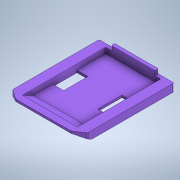
# Autodesk Inventor part: HullTop
Saved by Autodesk Inventor 2021 (Build 250183000, 183)
## iProperties
Created: 2021-05-14
Part Number: HullTop
Material: Generic
Document SubType Name: Modeling
Designer: ermoz
Density: 1 g/cm^3
Appearance: Default
Author: ermoz
Autodesk Inventor part; units mm, degrees
ref_plane "YZ Plane" through (0, 0, 0) normal (1, 0, 0) x (0, 1, 0)
ref_plane "XZ Plane" through (0, 0, 0) normal (0, 1, 0) x (-1, 0, 0)
ref_plane "XY Plane" through (0, 0, 0) normal (0, 0, 1) x (1, 0, 0)
sketch "Sketch1" plane through (0, 0, 0) normal (0, 1, 0) x (-1, 0, 0)
  line L0 (-34, 39.25) -> (34, 39.25)
  line L1 (34, 39.25) -> (34, -39.25)
  line L2 (34, -39.25) -> (-34, -39.25)
  line L3 (-34, -39.25) -> (-34, 39.25)
  line L4 (-34, 39.25) -> (34, -39.25) construction
  line L5 (34, 39.25) -> (-34, -39.25) construction
  line L6 (34, -39.25) -> (25, -39.25)
  line L7 (25, -39.25) -> (25, 39.25)
  line L8 (25, 39.25) -> (34, 39.25)
  line L9 (34, 39.25) -> (34, -39.25)
  line L10 (-34, -39.25) -> (-25, -39.25)
  line L11 (-25, -39.25) -> (-25, 39.25)
  line L12 (-25, 39.25) -> (-34, 39.25)
  line L13 (-34, 39.25) -> (-34, -39.25)
  circle A0 centre (29.5, 34.75) radius 1.5
  circle A1 centre (-29.5, 34.75) radius 1.5
  point P0 (0, 0)
  dimension "d0" = 78.5
  dimension "d1" = 68
  dimension "d2" = 9
  dimension "d3" = 9
  dimension "d4" = 3
  dimension "d5" = 4.5
  dimension "d6" = 3
  constraints: 28 end point, 6 parallel, 3 horizontal, 3 perpendicular, 2 centre point, 2 midpoint, 2 point on line
  measures "d0" distance of L0.end L1.end
  measures "d1" distance of L1.end L2.end
  measures "d2" distance of L7.end L8.end
  measures "d3" distance of L12.end L11.end
  measures "d4" diameter of A0
  measures "d5" distance from line of L0 A0.centre
  measures "d6" diameter of A1
extrude "Extrusion1" add sketch "Sketch1" along normal blind 2 contours L0 L7 L2 L11
extrude "Extrusion2" add sketch "Sketch1" along normal blind 7 contours L0 L11 L2 L3 | L0 L1 L2 L7 | A0 | A1
sketch "Sketch2" plane through (0, 2, 0) normal (0, 1, 0) x (1, 0, 0)
  line L0 (25, 39.25) -> (-25, 39.25) projected
  line L1 (-20, 39.25) -> (20, 39.25)
  line L2 (20, 39.25) -> (20, 36.25)
  line L3 (20, 36.25) -> (-20, 36.25)
  line L4 (-20, 36.25) -> (-20, 39.25)
  line L5 (25, 39.25) -> (25, -39.25) projected
  line L6 (-25, -39.25) -> (-25, 39.25) projected
  line L7 (-25, 39.25) -> (-20, 39.25)
  line L8 (-20, 39.25) -> (-20, 36.25)
  line L9 (-20, 36.25) -> (-25, 36.25)
  line L10 (-25, 36.25) -> (-25, 39.25)
  line L11 (20, 39.25) -> (25, 39.25)
  line L12 (25, 39.25) -> (25, 36.25)
  line L13 (25, 36.25) -> (20, 36.25)
  line L14 (20, 36.25) -> (20, 39.25)
  point P0 (0, 0)
  dimension "d11" = 3
  dimension "d12" = 5
  dimension "d13" = 5
  constraints: 24 end point, 6 parallel, 3 horizontal, 3 perpendicular, 3 point on line
  measures "d11" distance of L1.end L2.end
  measures "d12" distance between parallel lines of L5 L2
  measures "d13" distance between parallel lines of L6 L4
extrude "Extrusion3" add sketch "Sketch2" along normal up to surface (5 mm away) contours L5 L13 L2 L0 | L4 L9 L6 L0
extrude "Extrusion4" add sketch "Sketch2" along normal blind 9 contours L2 L3 L4 L0
sketch "Sketch5" plane through (0, 7, 0) normal (0, 1, 0) x (1, 0, 0)
  line L0 (-25, -39.25) -> (-25, 36.25) projected
  line L1 (-25, -39.25) -> (25, -39.25)
  line L2 (25, -39.25) -> (25, -45.25)
  line L3 (25, -45.25) -> (-25, -45.25)
  line L4 (-25, -45.25) -> (-25, -39.25)
  line L5 (-34, -39.25) -> (34, -39.25) projected
  line L6 (25, -45.25) -> (34, -39.25)
  line L7 (34, -39.25) -> (25, -39.25)
  line L8 (-34, 39.25) -> (-34, -39.25) projected
  line L9 (-25, -45.25) -> (-34, -39.25)
  line L10 (-34, -39.25) -> (-25, -39.25)
  point P0 (0, 0)
  dimension "d39" = 6
  constraints: 16 end point, 2 collinear, 2 parallel, 1 horizontal, 1 perpendicular
  measures "d39" distance of L1.end L2.end
extrude "Extrusion9" add sketch "Sketch5" against normal up to surface (7 mm away)
sketch "Sketch6" plane through (0, 0, 0) normal (0, -1, 0) x (1, 0, 0)
  line L0 (15, 11) -> (25, 11)
  line L1 (25, 11) -> (25, -11)
  line L2 (25, -11) -> (15, -11)
  line L3 (15, -11) -> (15, 11)
  line L4 (-25, -36.25) -> (-25, 39.25) projected
  line L5 (25, 39.25) -> (25, -36.25) projected
  line L6 (0, 0) -> (4.4691, 0)
  line L7 (-25, 11.8443) -> (-15, 11.8443)
  line L8 (-15, 11.8443) -> (-15, -10.1557)
  line L9 (-15, -10.1557) -> (-25, -10.1557)
  line L10 (-25, -10.1557) -> (-25, 11.8443)
  line L11 (-25, 11.8443) -> (-15, -10.1557) construction
  line L12 (-15, 11.8443) -> (-25, -10.1557) construction
  point P0 (-20, 0.8443)
  dimension "d42" = 10
  dimension "d43" = 22
  dimension "d54" = 10
  dimension "d55" = 22
  constraints: 22 end point, 4 parallel, 3 horizontal, 2 collinear, 2 midpoint, 2 perpendicular, 1 other
  measures "d42" distance of L0.start L0.end
  measures "d43" distance of L0.end L1.end
  measures "d54" distance of L8.end L9.end
  measures "d55" distance of L7.end L8.end
extrude "Extrusion10" cut sketch "Sketch6" against normal through all
chamfer "Chamfer1" distance 10 distance2 5 1 edges at (0, 2, 39.25) measured on face at (0, 2, 38.75)
chamfer "Chamfer2" distance 10 distance2 5 1 edges at (0, 0, 45.25) measured on face at (0, 0, 44.75)
fillet "Fillet2" radius 1 13 edges at (-34, 4.5, 39.25) (-25, 6, 45.25) (25, 6, 45.25) (34, 4.5, 39.25) (34, 3.5, -39.25) (-34, 3.5, -39.25) (0, 0, 35.25) (-20, 9, -39.25) (-20, 9, -36.25) (20, 9, -36.25) (20, 9, -39.25) (-25, 4.5, -36.25) (25, 4.5, -36.25)
body "Solid1"
